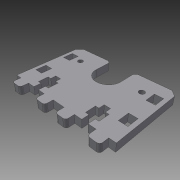
# Autodesk Inventor part: x_carriage_extruder_mount
Saved by Autodesk Inventor 2014 (Build 180170000, 170)
## iProperties
Created: 2013-11-28
Part Number: x_carriage_extruder_mount
Material: Generic
Document SubType Name: Modeling
Designer: buben
Density: 1 g/cm^3
Appearance: Default
Author: buben
Autodesk Inventor part; units mm, degrees
ref_plane "YZ Plane" through (0, 0, 0) normal (1, 0, 0) x (0, 1, 0)
ref_plane "XZ Plane" through (0, 0, 0) normal (0, 1, 0) x (-1, 0, 0)
ref_plane "XY Plane" through (0, 0, 0) normal (0, 0, 1) x (1, 0, 0)
sketch "Sketch1" plane through (0, 0, 0) normal (0, 0, 1) x (1, 0, 0)
  line L0 (0, 0) -> (80, 0)
  line L1 (80, 0) -> (80, 53)
  line L2 (0, 53) -> (0, 0)
  line L3 (30, 53) -> (30, 39)
  arc A0 (30, 39) -> (50, 39) centre (40, 39) ccw
  line L4 (50, 39) -> (50, 53)
  line L5 (80, 53) -> (50, 53)
  line L6 (30, 53) -> (0, 53)
  circle A1 centre (15, 39.5) radius 2.1
  circle A2 centre (65, 39.5) radius 2.1
  line L7 (3, 20) -> (9, 20)
  line L8 (9, 20) -> (9, 12)
  line L9 (9, 12) -> (3, 12)
  line L10 (3, 12) -> (3, 20)
  line L11 (71, 20) -> (77, 20)
  line L12 (77, 20) -> (77, 12)
  line L13 (77, 12) -> (71, 12)
  line L14 (71, 12) -> (71, 20)
  line L15 (71, 43) -> (77, 43)
  line L16 (77, 43) -> (77, 35)
  line L17 (77, 35) -> (71, 35)
  line L18 (71, 35) -> (71, 43)
  line L19 (3, 43) -> (9, 43)
  line L20 (9, 43) -> (9, 35)
  line L21 (9, 35) -> (3, 35)
  line L22 (3, 35) -> (3, 43)
  point P0 (40, 0)
  dimension "d0" = 80
  dimension "d1" = 53
  dimension "d2" = 20
  dimension "d3" = 14
  dimension "d4" = 13.5
  dimension "d5" = 4.2
  dimension "d6" = 4.2
  dimension "d9" = 8
  dimension "d10" = 6
  dimension "d11" = 8
  dimension "d12" = 15
  dimension "d13" = 3
  dimension "d14" = 12
  dimension "d15" = 8
  dimension "d16" = 8
  dimension "d17" = 6
  dimension "d18" = 3
  dimension "d19" = 50
  dimension "d20" = 15
  constraints: 46 end point, 13 parallel, 5 horizontal, 5 perpendicular, 5 vertical alignment, 3 centre point, 3 collinear, 2 point on circle, 2 tangent, 1 horizontal alignment, 1 midpoint
  measures "d0" distance of L0.start L0.end
  measures "d1" distance of L0.end L1.end
  measures "d2" distance between parallel lines of L4 L3
  measures "d3" distance of L4.start L4.end
  measures "d4" distance from line of L6 A1.centre
  measures "d5" diameter of A1
  measures "d6" diameter of A2
  measures "d9" distance of L21.end L19.start
  measures "d10" distance of L19.start L19.end
  measures "d11" distance of L9.end L7.start
  measures "d12" distance between parallel lines of L7 L21
  measures "d13" distance between parallel lines of L2 L22
  measures "d14" distance between parallel lines of L0 L9
  measures "d15" distance of L11.end L12.end
  measures "d16" distance of L15.end L16.end
  measures "d17" distance of L15.start L15.end
  measures "d18" distance between parallel lines of L1 L16
  measures "d19" distance of A2.centre A1.centre
  measures "d20" distance from line of L2 A1.centre
extrude "Extrusion1" add sketch "Sketch1" along normal blind 6
sketch "Sketch2" plane through (0, 0, 6) normal (0, 0, 1) x (1, 0, 0)
  line L0 (0, 0) -> (80, 0) projected
  line L1 (17.75, 16.3) -> (22.25, 16.3)
  line L2 (22.25, 0) -> (17.75, 0)
  line L3 (24.75, 12.3) -> (24.75, 5)
  line L4 (15.25, 5) -> (15.25, 12.3)
  line L5 (57.75, 16.3) -> (62.25, 16.3)
  line L6 (62.25, 0) -> (57.75, 0)
  line L7 (64.75, 12.3) -> (64.75, 5)
  line L8 (55.25, 5) -> (55.25, 12.3)
  line L9 (22.25, 16.3) -> (22.25, 12.3)
  line L10 (22.25, 5) -> (22.25, 0)
  line L11 (17.75, 0) -> (17.75, 5)
  line L12 (17.75, 12.3) -> (17.75, 16.3)
  line L13 (15.25, 12.3) -> (17.75, 12.3)
  line L14 (22.25, 12.3) -> (24.75, 12.3)
  line L15 (24.75, 5) -> (22.25, 5)
  line L16 (17.75, 5) -> (15.25, 5)
  line L17 (55.25, 12.3) -> (57.75, 12.3)
  line L18 (62.25, 12.3) -> (64.75, 12.3)
  line L19 (64.75, 5) -> (62.25, 5)
  line L20 (57.75, 5) -> (55.25, 5)
  line L21 (62.25, 16.3) -> (62.25, 12.3)
  line L22 (62.25, 5) -> (62.25, 0)
  line L23 (57.75, 0) -> (57.75, 5)
  line L24 (57.75, 12.3) -> (57.75, 16.3)
  line L25 (24.75, 8.65) -> (55.25, 8.65) construction
  point P0 (20, 16.3)
  point P1 (60, 16.3)
  point P2 (40, 8.65)
  point P3 (40, 0)
  dimension "d23" = 4.5
  dimension "d24" = 5
  dimension "d25" = 7.3
  dimension "d26" = 4
  dimension "d27" = 2.5
  dimension "d28" = 2.5
  dimension "d29" = 4.5
  dimension "d30" = 5
  dimension "d31" = 4
  dimension "d32" = 7.3
  dimension "d33" = 2.5
  dimension "d34" = 2.5
  dimension "d35" = 40
  constraints: 50 end point, 20 parallel, 10 collinear, 8 perpendicular, 6 horizontal, 6 midpoint, 1 vertical alignment
  measures "d23" distance of L1.start L1.end
  measures "d24" distance of L10.start L2.start
  measures "d25" distance of L3.start L3.end
  measures "d26" distance of L1.end L9.end
  measures "d27" distance of L9.end L3.start
  measures "d28" distance of L4.end L12.start
  measures "d29" distance of L5.start L5.end
  measures "d30" distance of L19.end L6.start
  measures "d31" distance of L5.end L18.start
  measures "d32" distance of L7.start L7.end
  measures "d33" distance of L18.start L7.start
  measures "d34" distance of L8.end L17.end
  measures "d35" distance of point (60, 16.3) point (20, 16.3)
extrude "Extrusion2" cut sketch "Sketch2" against normal through all
sketch "Sketch3" plane through (0, 0, 6) normal (0, 0, 1) x (1, 0, 0)
  line L0 (22.25, 0) -> (57.75, 0) projected
  line L1 (57.75, 16.3) -> (62.25, 16.3) projected
  line L2 (62.25, 0) -> (80, 0) projected
  line L3 (0, 0) -> (17.75, 0) projected
  line L4 (17.75, 16.3) -> (22.25, 16.3) projected
  line L5 (4.5, 0) -> (12.5, 0)
  line L6 (12.5, 0) -> (12.5, -4)
  line L7 (10.5, -6) -> (6.5, -6)
  line L8 (4.5, -4) -> (4.5, 0)
  line L9 (27.5, 0) -> (35.5, 0)
  line L10 (35.5, 0) -> (35.5, -4)
  line L11 (33.5, -6) -> (29.5, -6)
  line L12 (27.5, -4) -> (27.5, 0)
  line L13 (44.5, 0) -> (52.5, 0)
  line L14 (52.5, 0) -> (52.5, -4)
  line L15 (50.5, -6) -> (46.5, -6)
  line L16 (44.5, -4) -> (44.5, 0)
  line L17 (67.5, 0) -> (75.5, 0)
  line L18 (75.5, 0) -> (75.5, -4)
  line L19 (73.5, -6) -> (69.5, -6)
  line L20 (67.5, -4) -> (67.5, 0)
  arc A0 (4.5, -4) -> (6.5, -6) centre (6.5, -4) ccw
  arc A1 (10.5, -6) -> (12.5, -4) centre (10.5, -4) ccw
  arc A2 (27.5, -4) -> (29.5, -6) centre (29.5, -4) ccw
  arc A3 (33.5, -6) -> (35.5, -4) centre (33.5, -4) ccw
  arc A4 (44.5, -4) -> (46.5, -6) centre (46.5, -4) ccw
  arc A5 (50.5, -6) -> (52.5, -4) centre (50.5, -4) ccw
  arc A6 (67.5, -4) -> (69.5, -6) centre (69.5, -4) ccw
  arc A7 (73.5, -6) -> (75.5, -4) centre (73.5, -4) ccw
  point P0 (20, 16.3)
  point P1 (60, 16.3)
  dimension "d44" = 2
  dimension "d45" = 15
  dimension "d46" = 15
  dimension "d47" = 6
  dimension "d48" = 7.5
  dimension "d49" = 7.5
  dimension "d50" = 8
  dimension "d51" = 8
  dimension "d52" = 8
  dimension "d53" = 8
  constraints: 32 end point, 16 point on circle, 16 tangent, 8 centre point, 8 parallel, 7 equal radius, 4 horizontal, 4 perpendicular, 4 point on line, 3 collinear, 2 midpoint
  measures "d44" radius of A0
  measures "d45" distance between parallel lines of L12 L6
  measures "d46" distance between parallel lines of L20 L14
  measures "d47" distance between parallel lines of L3 L7
  measures "d48" distance from line of point (20, 16.3) L6
  measures "d49" distance from line of point (60, 16.3) L14
  measures "d50" distance between parallel lines of L6 L8
  measures "d51" distance between parallel lines of L10 L12
  measures "d52" distance between parallel lines of L14 L16
  measures "d53" distance between parallel lines of L18 L20
extrude "Extrusion3" add sketch "Sketch3" against normal blind 6
chamfer "Chamfer1" distance 4 angle 45 2 edges at (0, 53, 3) (80, 53, 3)
chamfer "Chamfer2" distance 2 angle 45 2 edges at (30, 53, 3) (50, 53, 3)
body "Solid1"
